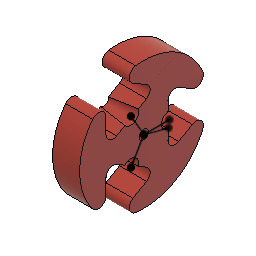
trinode (Autodesk Fusion 360 design; units mm, degrees)
Autodesk Fusion 360 part; units mm, degrees
sketch "Sketch1" plane through (0, 0, 0) normal (0, 1, 0) x (1, 0, 0)
sketch "Sketch2" plane through (0, 0, 0) normal (1, 0, 0) x (0, 0, -1)
  arc A0 (0.9551, -5.4164) -> (0.9551, 5.4164) centre (0, 0) ccw
  line L0 (0.9551, -5.4164) -> (0.9551, -12.7276)
  arc A1 (0.9551, -12.7276) -> (6.9551, -16.1918) centre (4.9551, -12.7276) ccw
  line L1 (6.9551, -16.1918) -> (16.5192, -10.6699)
  arc A2 (19.0192, -10) -> (16.5192, -10.6699) centre (19.0192, -15) ccw
  line L2 (19.0192, -10) -> (180.9808, -10)
  arc A3 (183.4808, -10.6699) -> (180.9808, -10) centre (180.9808, -15) ccw
  line L3 (183.4808, -10.6699) -> (193.0449, -16.1918)
  arc A4 (193.0449, -16.1918) -> (199.0449, -12.7276) centre (195.0449, -12.7276) ccw
  line L4 (199.0449, -12.7276) -> (199.0449, -5.4164)
  arc A5 (199.0449, 5.4164) -> (199.0449, -5.4164) centre (200, 0) ccw
  line L5 (199.0449, 5.4164) -> (199.0449, 12.7276)
  arc A6 (199.0449, 12.7276) -> (193.0449, 16.1918) centre (195.0449, 12.7276) ccw
  line L6 (193.0449, 16.1918) -> (183.4808, 10.6699)
  arc A7 (180.9808, 10) -> (183.4808, 10.6699) centre (180.9808, 15) ccw
  line L7 (180.9808, 10) -> (19.0192, 10)
  arc A8 (16.5192, 10.6699) -> (19.0192, 10) centre (19.0192, 15) ccw
  line L8 (16.5192, 10.6699) -> (6.9551, 16.1918)
  arc A9 (6.9551, 16.1918) -> (0.9551, 12.7276) centre (4.9551, 12.7276) ccw
  line L9 (0.9551, 12.7276) -> (0.9551, 5.4164)
  line L10 (6.9551, 16.1918) -> (16.0862, 10.9199)
  arc A10 (16.0862, 10.9199) -> (23.4826, 17.4411) centre (18.6872, 15.4249) ccw
  arc A11 (-22.7868, 19.1238) -> (-32.1683, 13.7073) centre (-27, 15.5885) ccw
  arc A12 (-44.5, 13.5158) -> (-38.5, 10.0517) centre (-40.5, 13.5158) ccw
  line L11 (-44.5, 13.5158) -> (-44.5, 24.0596)
  line L12 (-38.5, 10.0517) -> (-32.1683, 13.7073)
  line L13 (-22.7868, 19.1238) -> (-16.4551, 22.7794)
  arc A13 (-16.4551, 22.7794) -> (-16.4551, 29.7076) centre (-18.4551, 26.2435) ccw
  line L14 (-16.4551, 29.7076) -> (-26.0192, 35.2295)
  arc A14 (-32.1683, -13.7073) -> (-22.7868, -19.1238) centre (-27, -15.5885) ccw
  arc A15 (-16.4551, -29.7076) -> (-16.4551, -22.7794) centre (-18.4551, -26.2435) ccw
  line L15 (-16.4551, -29.7076) -> (-25.5862, -34.9795)
  line L16 (-16.4551, -22.7794) -> (-22.7868, -19.1238)
  line L17 (-32.1683, -13.7073) -> (-38.5, -10.0517)
  arc A16 (-38.5, -10.0517) -> (-44.5, -13.5158) centre (-40.5, -13.5158) ccw
  line L18 (-44.5, -13.5158) -> (-44.5, -24.5596)
  line L19 (-18, 0) -> (4.5, 38.9711)
  line L20 (-18, 0) -> (27, 0) construction
  line L21 (6.9551, 16.1918) -> (6.5221, 16.4418)
  arc A17 (6.5221, 16.4418) -> (-0.9551, 12.1248) centre (4.0297, 12.1248) ccw
  line L22 (-0.9551, 12.1248) -> (-0.9551, 5.4164)
  arc A18 (-0.9551, 5.4164) -> (-5.5, 0) centre (0, 0) ccw
  arc A19 (23.4826, 17.4411) -> (4.5, 38.9711) centre (-18, 0) ccw
  line L23 (-18, 0) -> (4.5, -38.9711)
  arc A20 (-5.5, 0) -> (-0.9551, -5.4164) centre (0, 0) ccw
  line L24 (-0.9551, -12.1248) -> (-0.9551, -5.4164)
  arc A21 (-0.9551, -12.1248) -> (6.5221, -16.4418) centre (4.0297, -12.1248) ccw
  line L25 (6.9551, -16.1918) -> (6.5221, -16.4418)
  line L26 (6.9551, -16.1918) -> (16.0862, -10.9199)
  arc A22 (23.4826, -17.4411) -> (16.0862, -10.9199) centre (18.6872, -15.4249) ccw
  arc A23 (4.5, -38.9711) -> (23.4826, -17.4411) centre (-18, 0) ccw
  circle A24 centre (0, 0) radius 5.5
  line L27 (-0.9551, 5.4164) -> (-0.9551, -5.4164)
  point P0 (-18, 0)
  dimension "d31" = 0.5
  dimension "d32" = 18
  dimension "d34" = 360
  dimension "d35" = 20.1035
  dimension "d36" = 20
  dimension "d37" = 12.3332
  dimension "d41" = 60
  dimension "d42" = 0.5
  dimension "d43" = 45
  constraint coincident L8.end A9.start
  constraint coincident L8 L10.end
  constraint parallel L8 L10
  constraint tangent L10 A10
  constraint horizontal P0 A0.centre
  constraint coincident P0 L19.start
  constraint horizontal L20
  constraint equal L19 L20
  constraint tangent A9 L21
  constraint tangent L21 A17
  constraint parallel L9 L22
  constraint tangent A17 L22
  constraint coincident A0.centre A18.centre
  constraint coincident L20 A18.end
  constraint horizontal A0.end L22.end
  constraint equal A0 A18
  constraint tangent A10 A19
  constraint coincident L19.end A19.end
  constraint symmetric L8.end L20 A1.end
  constraint symmetric L10.end L20 L26.end
  constraint symmetric A10.end L20 A22.start
  constraint symmetric A10 L20 A22
  constraint symmetric P0 L20 L19.start
  constraint symmetric L19.end L20 L23.end
  constraint symmetric L20 L8.end A1.end
  constraint symmetric L20 L21.end A21.end
  constraint symmetric L20 A17.end L24.start
  constraint symmetric L20 A17 A21
  constraint symmetric L20 L22.end A20.end
  constraint symmetric L20 A18.end A20.start
  constraint symmetric L20 A18 A20
  constraint symmetric L20 L19.end L23.end
  constraint symmetric L20 A19 A23
  constraint concentric A0 A24
  constraint coincident L22.end A24
  measures "d31" distance of A8.start L10.end
  measures "d32" distance of P0 A0.centre
  measures "d35" distance of A9.end L13.end
  measures "d36" distance of A2.start L7.end
  measures "d37" distance of A0.end L8.end
  measures "d41" angle of L19 L20
  measures "d42" distance of L8.end L21.end
  measures "d43" radius of A19
extrude "Extrude1" add sketch "Sketch2" against normal blind 19 contours L1 L8 L10 A10 L19 L21 A17 L22 A18 A19 L23 A20 L24 A21 L25 L26 A22 A23 A24 | A18 A20 A24 L27 makes body 1
extrude "Extrude2" cut sketch "Sketch2" against normal up to surface (19 mm away) draft -6.6 contours A0 A24 L27 | A18 A20 A24 L27 bodies 1
pattern_circular "C-Pattern1" count 3 over 360 about axis through (0, 0, 18) along (-1, 0, 0) of bodies 1 makes body 2 at (-19, -20.6497, 9.1744) makes body 3 at (-19, 20.6497, 9.1744)
combine "Combine1" operation add target body 1 tool bodies 3 2
sketch "Sketch3" plane through (0, 0, 0) normal (1, 0, 0) x (0, 0, -1)
  arc A0 (-0.9551, 5.4164) -> (-0.9551, -5.4164) centre (0, 0) ccw
  line L0 (-0.9551, 5.4164) -> (-0.9551, 12.1248)
  arc A1 (6.5221, 16.4418) -> (-0.9551, 12.1248) centre (4.0297, 12.1248) ccw
  line L1 (6.5221, 16.4418) -> (16.0862, 10.9199)
  arc A2 (16.0862, 10.9199) -> (23.4826, 17.4411) centre (18.6872, 15.4249) ccw
  arc A3 (23.4826, 17.4411) -> (-23.6368, 44.6456) centre (-18, 0) ccw
  arc A4 (-23.6368, 44.6456) -> (-25.5862, 34.9795) centre (-22.9852, 39.4845) ccw
  line L2 (-25.5862, 34.9795) -> (-16.0221, 29.4576)
  arc A5 (-16.0221, 20.8238) -> (-16.0221, 29.4576) centre (-18.5144, 25.1407) ccw
  line L3 (-16.0221, 20.8238) -> (-21.8317, 17.4696)
  arc A6 (-31.2132, 12.0531) -> (-21.8317, 17.4696) centre (-27, 15.5885) ccw
  line L4 (-31.2132, 12.0531) -> (-37.0229, 8.6989)
  arc A7 (-44.5, 13.0158) -> (-37.0229, 8.6989) centre (-39.5153, 13.0158) ccw
  line L5 (-44.5, 13.0158) -> (-44.5, 24.0596)
  arc A8 (-44.5, 24.0596) -> (-53.8458, 27.2044) centre (-49.702, 24.0596) ccw
  arc A9 (-53.8458, 27.2044) -> (-53.8458, -27.2044) centre (-18, 0) ccw
  arc A10 (-53.8458, -27.2044) -> (-44.5, -24.0596) centre (-49.702, -24.0596) ccw
  line L6 (-44.5, -24.0596) -> (-44.5, -13.0158)
  arc A11 (-37.0229, -8.6989) -> (-44.5, -13.0158) centre (-39.5153, -13.0158) ccw
  line L7 (-37.0229, -8.6989) -> (-31.2132, -12.0531)
  arc A12 (-21.8317, -17.4696) -> (-31.2132, -12.0531) centre (-27, -15.5885) ccw
  line L8 (-21.8317, -17.4696) -> (-16.0221, -20.8238)
  arc A13 (-16.0221, -29.4576) -> (-16.0221, -20.8238) centre (-18.5144, -25.1407) ccw
  line L9 (-16.0221, -29.4576) -> (-25.5862, -34.9795)
  arc A14 (-25.5862, -34.9795) -> (-23.6368, -44.6456) centre (-22.9852, -39.4845) ccw
  arc A15 (-23.6368, -44.6456) -> (23.4826, -17.4411) centre (-18, 0) ccw
  arc A16 (23.4826, -17.4411) -> (16.0862, -10.9199) centre (18.6872, -15.4249) ccw
  line L10 (16.0862, -10.9199) -> (6.5221, -16.4418)
  arc A17 (-0.9551, -12.1248) -> (6.5221, -16.4418) centre (4.0297, -12.1248) ccw
  line L11 (-0.9551, -12.1248) -> (-0.9551, -5.4164)
  circle A18 centre (-18, 0) radius 3.25
  dimension "d50" = 6.5
  constraint concentric A3 A18
  measures "d50" diameter of A18
extrude "Extrude3" cut sketch "Sketch3" against normal up to surface (19 mm away) contours A18 bodies 1
sketch "Sketch5" plane through (0, 0, 0) normal (1, 0, 0) x (0, 0, -1)
  circle A0 centre (-18, 0) radius 3.25
  arc A1 (-0.9551, 5.4164) -> (-0.9551, -5.4164) centre (0, 0) ccw
  line L0 (-0.9551, 5.4164) -> (-0.9551, 12.1248)
  arc A2 (6.5221, 16.4418) -> (-0.9551, 12.1248) centre (4.0297, 12.1248) ccw
  line L1 (6.5221, 16.4418) -> (16.0862, 10.9199)
  arc A3 (16.0862, 10.9199) -> (23.4826, 17.4411) centre (18.6872, 15.4249) ccw
  arc A4 (23.4826, 17.4411) -> (-23.6368, 44.6456) centre (-18, 0) ccw
  arc A5 (-23.6368, 44.6456) -> (-25.5862, 34.9795) centre (-22.9852, 39.4845) ccw
  line L2 (-25.5862, 34.9795) -> (-16.0221, 29.4576)
  arc A6 (-16.0221, 20.8238) -> (-16.0221, 29.4576) centre (-18.5144, 25.1407) ccw
  line L3 (-16.0221, 20.8238) -> (-21.8317, 17.4696)
  arc A7 (-31.2132, 12.0531) -> (-21.8317, 17.4696) centre (-27, 15.5885) ccw
  line L4 (-31.2132, 12.0531) -> (-37.0229, 8.6989)
  arc A8 (-44.5, 13.0158) -> (-37.0229, 8.6989) centre (-39.5153, 13.0158) ccw
  line L5 (-44.5, 13.0158) -> (-44.5, 24.0596)
  arc A9 (-44.5, 24.0596) -> (-53.8458, 27.2044) centre (-49.702, 24.0596) ccw
  arc A10 (-53.8458, 27.2044) -> (-53.8458, -27.2044) centre (-18, 0) ccw
  arc A11 (-53.8458, -27.2044) -> (-44.5, -24.0596) centre (-49.702, -24.0596) ccw
  line L6 (-44.5, -24.0596) -> (-44.5, -13.0158)
  arc A12 (-37.0229, -8.6989) -> (-44.5, -13.0158) centre (-39.5153, -13.0158) ccw
  line L7 (-37.0229, -8.6989) -> (-31.2132, -12.0531)
  arc A13 (-21.8317, -17.4696) -> (-31.2132, -12.0531) centre (-27, -15.5885) ccw
  line L8 (-21.8317, -17.4696) -> (-16.0221, -20.8238)
  arc A14 (-16.0221, -29.4576) -> (-16.0221, -20.8238) centre (-18.5144, -25.1407) ccw
  line L9 (-16.0221, -29.4576) -> (-25.5862, -34.9795)
  arc A15 (-25.5862, -34.9795) -> (-23.6368, -44.6456) centre (-22.9852, -39.4845) ccw
  arc A16 (-23.6368, -44.6456) -> (23.4826, -17.4411) centre (-18, 0) ccw
  arc A17 (23.4826, -17.4411) -> (16.0862, -10.9199) centre (18.6872, -15.4249) ccw
  line L10 (16.0862, -10.9199) -> (6.5221, -16.4418)
  arc A18 (-0.9551, -12.1248) -> (6.5221, -16.4418) centre (4.0297, -12.1248) ccw
  line L11 (-0.9551, -12.1248) -> (-0.9551, -5.4164)
  line L12 (-18, 0) -> (0, 0)
  line L13 (-18, 0) -> (-27, 15.5885)
  line L14 (-18, 0) -> (-27, -15.5885)
  line L15 (-18, 0) -> (-0.6133, -4.6587)
  dimension "d5" = 15
  constraint coincident A0.centre A4.centre
  constraint horizontal L12
  constraint coincident A7.centre L13.end
  constraint coincident A13.centre L14.end
  constraint equal L12 L14
  constraint equal L12 L15
  measures "d5" angle of L12 L15
sketch "Sketch4" plane through (0, 0, 0) normal (1, 0, 0) x (0, 0, -1)
  circle A0 centre (-18, 0) radius 3.25
  arc A1 (-0.9551, 5.4164) -> (-0.9551, -5.4164) centre (0, 0) ccw
  line L0 (-0.9551, 5.4164) -> (-0.9551, 12.1248)
  arc A2 (6.5221, 16.4418) -> (-0.9551, 12.1248) centre (4.0297, 12.1248) ccw
  line L1 (6.5221, 16.4418) -> (16.0862, 10.9199)
  arc A3 (16.0862, 10.9199) -> (23.4826, 17.4411) centre (18.6872, 15.4249) ccw
  arc A4 (23.4826, 17.4411) -> (-23.6368, 44.6456) centre (-18, 0) ccw
  arc A5 (-23.6368, 44.6456) -> (-25.5862, 34.9795) centre (-22.9852, 39.4845) ccw
  line L2 (-25.5862, 34.9795) -> (-16.0221, 29.4576)
  arc A6 (-16.0221, 20.8238) -> (-16.0221, 29.4576) centre (-18.5144, 25.1407) ccw
  line L3 (-16.0221, 20.8238) -> (-21.8317, 17.4696)
  arc A7 (-31.2132, 12.0531) -> (-21.8317, 17.4696) centre (-27, 15.5885) ccw
  line L4 (-31.2132, 12.0531) -> (-37.0229, 8.6989)
  arc A8 (-44.5, 13.0158) -> (-37.0229, 8.6989) centre (-39.5153, 13.0158) ccw
  line L5 (-44.5, 13.0158) -> (-44.5, 24.0596)
  arc A9 (-44.5, 24.0596) -> (-53.8458, 27.2044) centre (-49.702, 24.0596) ccw
  arc A10 (-53.8458, 27.2044) -> (-53.8458, -27.2044) centre (-18, 0) ccw
  arc A11 (-53.8458, -27.2044) -> (-44.5, -24.0596) centre (-49.702, -24.0596) ccw
  line L6 (-44.5, -24.0596) -> (-44.5, -13.0158)
  arc A12 (-37.0229, -8.6989) -> (-44.5, -13.0158) centre (-39.5153, -13.0158) ccw
  line L7 (-37.0229, -8.6989) -> (-31.2132, -12.0531)
  arc A13 (-21.8317, -17.4696) -> (-31.2132, -12.0531) centre (-27, -15.5885) ccw
  line L8 (-21.8317, -17.4696) -> (-16.0221, -20.8238)
  arc A14 (-16.0221, -29.4576) -> (-16.0221, -20.8238) centre (-18.5144, -25.1407) ccw
  line L9 (-16.0221, -29.4576) -> (-25.5862, -34.9795)
  arc A15 (-25.5862, -34.9795) -> (-23.6368, -44.6456) centre (-22.9852, -39.4845) ccw
  arc A16 (-23.6368, -44.6456) -> (23.4826, -17.4411) centre (-18, 0) ccw
  arc A17 (23.4826, -17.4411) -> (16.0862, -10.9199) centre (18.6872, -15.4249) ccw
  line L10 (16.0862, -10.9199) -> (6.5221, -16.4418)
  arc A18 (-0.9551, -12.1248) -> (6.5221, -16.4418) centre (4.0297, -12.1248) ccw
  line L11 (-0.9551, -12.1248) -> (-0.9551, -5.4164)
  line L12 (-13.5297, 45) -> (-63, 45)
  line L13 (-63, 45) -> (-63, -45)
  line L14 (-63, -45) -> (-13.5297, -45)
  line L15 (-13.5297, -45) -> (-13.5297, 45)
  constraint horizontal L12
  constraint vertical L13
  constraint horizontal L14
  constraint vertical L15
  constraint tangent A10 L13
  constraint tangent A4 L12
  constraint tangent A16 L14
  constraint tangent A6 L15
extrude "Extrude4" [suppressed]
extrude "Extrude5" [suppressed]
